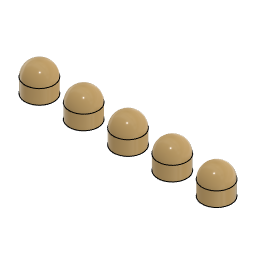
Stand Off Isolator (Printable) (Autodesk Fusion 360 design; units mm, degrees)
Autodesk Fusion 360 part; units mm, degrees
sketch "post void" plane through (0, 0, 0) normal (0, 0, 1) x (1, 0, 0)
  circle A0 centre (0, 0) radius 3.75
  line L0 (0, 0) -> (1.875, 3.2476)
  line L1 (0, 0) -> (3.75, 0) construction
  line L2 (0, 0) -> (-1.875, 3.2476)
  line L3 (0, 0) -> (-3.75, 0)
  line L4 (0, 0) -> (-1.875, -3.2476)
  line L5 (0, 0) -> (1.875, -3.2476)
  line L6 (0, 0) -> (3.75, 0)
  line L7 (3.75, 0) -> (1.875, -3.2476)
  line L8 (1.875, -3.2476) -> (-1.875, -3.2476)
  line L9 (-1.875, -3.2476) -> (-3.75, 0)
  line L10 (-3.75, 0) -> (-1.875, 3.2476)
  line L11 (-1.875, 3.2476) -> (1.875, 3.2476)
  line L12 (1.875, 3.2476) -> (3.75, 0)
  dimension "d32" = 7.5
  dimension "d34" = 60
  dimension "d35" = 3.75
  dimension "d36" = 60
  dimension "d37" = 3.75
  dimension "d38" = 60
  dimension "d39" = 3.75
  dimension "d40" = 60
  dimension "d41" = 3.75
  dimension "d42" = 60
  dimension "d43" = 3.75
  dimension "d44" = 60
  dimension "d45" = 3.75
  constraint coincident A0.centre L0.start
  constraint horizontal L1
  constraint parallel L0 L7
  measures "d32" diameter of A0
  measures "d34" angle of L0 L1
  measures "d35" distance of A0.centre L0.end
  measures "d36" angle of L0 L2
  measures "d37" distance of A0.centre L2.end
  measures "d38" angle of L2 L3
  measures "d39" distance of A0.centre L3.end
  measures "d40" angle of L3 L4
  measures "d41" distance of A0.centre L4.end
  measures "d42" angle of L4 L5
  measures "d43" distance of A0.centre L5.end
  measures "d44" angle of L5 L6
  measures "d45" distance of A0.centre L1.end
sketch "Sketch4" plane through (0, 0, 0) normal (0, 0, 1) x (1, 0, 0)
  line L0 (3.75, 0) -> (4.75, 0)
  line L1 (4.75, 0) -> (5.75, 0)
  circle A0 centre (0, 0) radius 4.75
  circle A1 centre (0, 0) radius 5.75
  dimension "d56" = 1
  dimension "d57" = 1
  constraint horizontal L0
  constraint parallel L0 L1
  constraint coincident A0.centre A1.centre
  constraint coincident L0.end A0
  constraint concentric A0 A1
  constraint coincident L1.end A1
  measures "d56" distance of L0.start L0.end
  measures "d57" distance of L0.end L1.end
sketch "Wall" plane through (0, 0, 0) normal (0, 0, 1) x (1, 0, 0)
  circle A0 centre (0, 0) radius 6.5
  dimension "d46" = 13
  constraint coincident A0.centre origin
  measures "d46" diameter of A0
extrude "Extrude1" add sketch "Wall" along normal blind 13 makes body 1
extrude "Extrude2" cut sketch "post void" along normal blind 8 contours L5 L6 L7 | L0 L6 L12 | L0 L2 L11 | L4 L5 L8 | L2 L3 L10 | L3 L4 L9 bodies 1
sketch "Sketch3" plane through (0, 0, 0) normal (0, 0, 1) x (1, 0, 0)
  circle A0 centre (0, 0) radius 2.25
  dimension "d51" = 4.5
  constraint coincident A0.centre origin
  measures "d51" diameter of A0
extrude "Extrude3" cut sketch "Sketch3" along normal blind 10 bodies 1
fillet "Fillet1" radius 6.5 1 edges at (-6.0601, -2.3505, 13) on bodies 1
copy_body "CopyPasteBodies3" bodies 1 makes body 2
move_body "Move3" bodies 2 to x (1, 0, 0) y (0, 1, 0) z (0, 0, 1) at (20, 0, 0)
copy_body "CopyPasteBodies4" bodies 1 makes body 3
move_body "Move4" bodies 3 to x (1, 0, 0) y (0, 1, 0) z (0, 0, 1) at (40, 0, 0)
copy_body "CopyPasteBodies5" bodies 1 makes body 4
move_body "Move5" bodies 4 to x (1, 0, 0) y (0, 1, 0) z (0, 0, 1) at (60, 0, 0)
copy_body "CopyPasteBodies6" bodies 1 makes body 5
move_body "Move6" bodies 5 to x (1, 0, 0) y (0, 1, 0) z (0, 0, 1) at (80, 0, 0)
equation "d35 = ( 7.5 / 2 ) * 1 mm"
equation "d37 = ( 7.5 / 2 ) * 1 mm"
equation "d39 = ( 7.5 / 2 ) * 1 mm"
equation "d41 = ( 7.5 / 2 ) * 1 mm"
equation "d43 = ( 7.5 / 2 ) * 1 mm"
equation "d45 = ( 7.5 / 2 ) * 1 mm"
equation "d47 = 11 mm + 2 mm"
equation "d49 = 10.00 mm - 2 mm"
named bodies: "Sketch Body", "13mm", "2.75 body + 0.5 head", "13mm (1)", "2.75 Body + 1.0 head", "13mm (2)", "2.75 Body + 2.0 head", "2.75 Body + 3.0 head"
